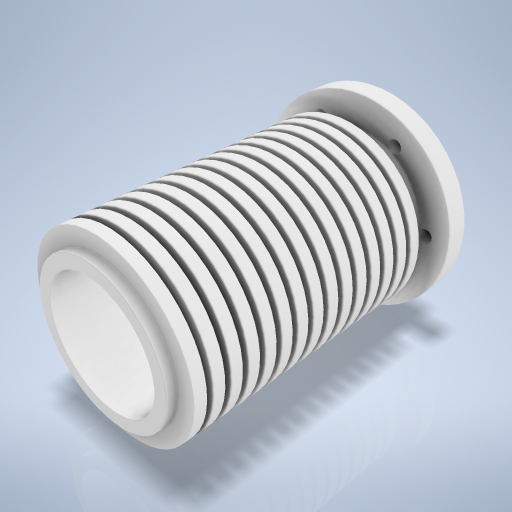
# Autodesk Inventor part: 14
Saved by Autodesk Inventor 2024.2 (Build 282272000, 272)
## iProperties
Created: 2024-05-05
Part Number: 14
Material: PBT-Kunststoff
Document SubType Name: Modeling
Designer: Fabri
Density: 1.31 g/cm^3
Appearance: Glatt - Weiß
Author: Fabri
Autodesk Inventor part; units mm, degrees
ref_plane "XZ Plane" through (0, 0, 0) normal (0, 1, 0) x (-1, 0, 0)
ref_plane "XY Plane" through (0, 0, 0) normal (0, 0, 1) x (1, 0, 0)
sketch "Skizze1" plane through (0, 0, 0) normal (0, 1, 0) x (-1, 0, 0)
  circle A0 centre (0, 0) radius 55
  dimension "d0" = 110
  constraints: 1 centre point, 1 coincident
  measures "d0" diameter of A0
extrude "Extrusion1" add sketch "Skizze1" along normal blind 235
ref_plane "Arbeitsebene1" through (0, 0, 0) normal (1, 0, 0) x (0, 1, 0)
sketch "Skizze2" plane through (0, 0, 0) normal (1, 0, 0) x (0, 1, 0)
  line L0 (235, -55) -> (235, 55) projected
  line L1 (0, -55) -> (0, 55) projected
  line L2 (0, -55) -> (235, -55) projected
  line L3 (0, 55) -> (235, 55) projected
  line L4 (7, -55) -> (7, -67.5)
  line L5 (7, -67.5) -> (15.5, -67.5)
  line L6 (15.5, -67.5) -> (15.5, -55)
  line L7 (0, 0) -> (235, 0)
  line L8 (28, -67.5) -> (28, -55)
  line L9 (19.5, -55) -> (19.5, -67.5)
  line L10 (19.5, -67.5) -> (28, -67.5)
  line L11 (40.5, -67.5) -> (40.5, -55)
  line L12 (32, -55) -> (32, -67.5)
  line L13 (32, -67.5) -> (40.5, -67.5)
  line L14 (53, -67.5) -> (53, -55)
  line L15 (44.5, -55) -> (44.5, -67.5)
  line L16 (44.5, -67.5) -> (53, -67.5)
  line L17 (65.5, -67.5) -> (65.5, -55)
  line L18 (57, -55) -> (57, -67.5)
  line L19 (57, -67.5) -> (65.5, -67.5)
  line L20 (78, -67.5) -> (78, -55)
  line L21 (69.5, -55) -> (69.5, -67.5)
  line L22 (69.5, -67.5) -> (78, -67.5)
  line L23 (90.5, -67.5) -> (90.5, -55)
  line L24 (82, -55) -> (82, -67.5)
  line L25 (82, -67.5) -> (90.5, -67.5)
  line L26 (103, -67.5) -> (103, -55)
  line L27 (94.5, -55) -> (94.5, -67.5)
  line L28 (94.5, -67.5) -> (103, -67.5)
  line L29 (115.5, -67.5) -> (115.5, -55)
  line L30 (107, -55) -> (107, -67.5)
  line L31 (107, -67.5) -> (115.5, -67.5)
  line L32 (128, -67.5) -> (128, -55)
  line L33 (119.5, -55) -> (119.5, -67.5)
  line L34 (119.5, -67.5) -> (128, -67.5)
  line L35 (140.5, -67.5) -> (140.5, -55)
  line L36 (132, -55) -> (132, -67.5)
  line L37 (132, -67.5) -> (140.5, -67.5)
  line L38 (153, -67.5) -> (153, -55)
  line L39 (144.5, -55) -> (144.5, -67.5)
  line L40 (144.5, -67.5) -> (153, -67.5)
  line L41 (165.5, -67.5) -> (165.5, -55)
  line L42 (157, -55) -> (157, -67.5)
  line L43 (157, -67.5) -> (165.5, -67.5)
  line L44 (178, -67.5) -> (178, -55)
  line L45 (169.5, -55) -> (169.5, -67.5)
  line L46 (169.5, -67.5) -> (178, -67.5)
  line L47 (190.5, -67.5) -> (190.5, -55)
  line L48 (182, -55) -> (182, -67.5)
  line L49 (182, -67.5) -> (190.5, -67.5)
  line L50 (190.5, -55) -> (182, -55)
  line L51 (178, -55) -> (169.5, -55)
  line L52 (165.5, -55) -> (157, -55)
  line L53 (153, -55) -> (144.5, -55)
  line L54 (140.5, -55) -> (132, -55)
  line L55 (128, -55) -> (119.5, -55)
  line L56 (115.5, -55) -> (107, -55)
  line L57 (103, -55) -> (94.5, -55)
  line L58 (90.5, -55) -> (82, -55)
  line L59 (78, -55) -> (69.5, -55)
  line L60 (65.5, -55) -> (57, -55)
  line L61 (53, -55) -> (44.5, -55)
  line L62 (40.5, -55) -> (32, -55)
  line L63 (28, -55) -> (19.5, -55)
  line L64 (15.5, -55) -> (7, -55)
  line L65 (208, -55) -> (208, -77.5)
  line L66 (208, -77.5) -> (224, -77.5)
  line L67 (224, -77.5) -> (224, -55)
  line L68 (208, -55) -> (224, -55)
  point P0 (7, -61.25)
  point P1 (19.5, -61.25)
  point P2 (32, -61.25)
  point P3 (44.5, -61.25)
  point P4 (57, -61.25)
  point P5 (69.5, -61.25)
  point P6 (82, -61.25)
  point P7 (94.5, -61.25)
  point P8 (107, -61.25)
  point P9 (119.5, -61.25)
  point P10 (132, -61.25)
  point P11 (144.5, -61.25)
  point P12 (157, -61.25)
  point P13 (169.5, -61.25)
  point P14 (182, -61.25)
  point P15 (190.5, -55)
  point P16 (178, -55)
  point P17 (165.5, -55)
  point P18 (153, -55)
  point P19 (140.5, -55)
  point P20 (128, -55)
  point P21 (115.5, -55)
  point P22 (103, -55)
  point P23 (90.5, -55)
  point P24 (78, -55)
  point P25 (65.5, -55)
  point P26 (53, -55)
  point P27 (40.5, -55)
  point P28 (28, -55)
  dimension "d4" = 7
  dimension "d5" = 8.5
  dimension "d6" = 135
  dimension "d9" = 12.5
  dimension "d15" = 16
  dimension "d16" = 11
  dimension "d17" = 155
  constraints: 130 end point, 70 horizontal alignment, 28 parallel, 17 horizontal, 14 collinear, 3 vertical, 2 midpoint, 2 perpendicular, 5 other
  measures "d4" distance from line of L1 point (7, -61.25)
  measures "d5" distance between parallel lines of L4 L6
  measures "d6" diameter of L5 L7
  measures "d9" distance of L5.end L8.start
  measures "d15" distance between parallel lines of L65 L67
  measures "d16" distance between parallel lines of L67 L0
  measures "d17" diameter of L66 L7
revolve "Umdrehung1" add sketch "Skizze2" angle 360 about axis through (0, 0, 0) along (0, 1, 0) contours L67 L66 L65 L2 | L47 L49 L48 L2 | L2 L6 L5 L4 | L44 L46 L45 L2 | L2 L8 L10 L9 | L41 L43 L42 L2 | L2 L11 L13 L12 | L38 L40 L39 L2 | L2 L14 L16 L15 | L35 L37 L36 L2 | L2 L17 L19 L18 | L32 L34 L33 L2 | L2 L20 L22 L21 | L29 L31 L30 L2 | L2 L23 L25 L24 | L26 L28 L27 L2
sketch "Skizze3" plane through (0, 235, 0) normal (0, 1, 0) x (1, 0, 0)
  circle A0 centre (0, 0) radius 55 projected
  constraints: 1 coincident
hole "Bohrung1" at (0, 235, 0) direction (0, -1, 0) diameter 90 depth 235
sketch "Skizze4" plane through (0, 224, 0) normal (0, 1, 0) x (1, 0, 0)
  circle A0 centre (0, 0) radius 60 construction
  line L0 (0, 0) -> (-44.5912, -77.2343) construction
  circle A1 centre (0, 0) radius 55 projected
  line L1 (0, 0) -> (43.5598, -75.4477) construction
  line L2 (0, 0) -> (0, -79.8466) construction
  point P0 (-30, -51.9615)
  dimension "d25" = 120
  dimension "d26" = 60
  dimension "d27" = 30
  constraints: 6 end point, 1 coincident, 1 point on line, 1 vertical, 3 other
  measures "d26" angle of L0 L1
  measures "d27" angle of L0 L2
hole "Bohrung2" at (-30, 224, 51.9615) direction (0, -1, 0) diameter 10 depth 16
pattern_circular "Runde Anordnung1" count 6 over 360 about axis through (0, 216, 0) along (0, 1, 0) of "Bohrung2"
